skadis_nut_coupon (Autodesk Fusion 360 design; units mm, degrees)
part number: 2026-09-06-14-40-16-018
Autodesk Fusion 360 part; units mm, degrees
sketch "Plate" plane through (0, 0, 0) normal (0, 1, 0) x (1, 0, 0)
  line L0 (0, 0) -> (11, 0)
  line L1 (11, 0) -> (11, -20)
  line L2 (11, -20) -> (0, -20)
  line L3 (0, -20) -> (0, 0)
  dimension "d64" = 11
  dimension "d65" = 20
  constraint coincident L0.start L3.end
  constraint horizontal L0
  constraint horizontal L2
  constraint vertical L1
  constraint vertical L3
  measures "d64" horizontal distance of L0.start L1.end
  measures "d65" vertical distance of L0.start L1.end
extrude "Plate (1)" add sketch "Plate" along normal mid plane 33 from surface at 4.5
sketch "Screw hole" plane through (0, 0, 0) normal (0, 1, 0) x (1, 0, 0)
  line L0 (-1, -7.6) -> (12, -7.6)
  line L1 (12, -7.6) -> (12, -12.4)
  line L2 (12, -12.4) -> (-1, -12.4)
  line L3 (-1, -12.4) -> (-1, -7.6)
  dimension "d69" = 12
  dimension "d70" = 7.6
  dimension "d71" = 13
  dimension "d72" = 4.8
  constraint horizontal L0
  constraint horizontal L2
  constraint vertical L1
  constraint vertical L3
  measures "d69" horizontal distance of origin L0.end
  measures "d70" vertical distance of origin L0.end
  measures "d71" horizontal distance of L0.start L0.end
  measures "d72" vertical distance of L0.end L1.end
extrude "Screw hole (1)" cut sketch "Screw hole" along normal mid plane 16.8 from surface at 7.52
sketch "Nut cavity" plane through (0, 0, 0) normal (0, 1, 0) x (1, 0, 0)
  line L0 (5.5, -6.3) -> (8, -6.3)
  line L1 (8, -6.3) -> (8, -13.7)
  line L2 (8, -13.7) -> (5.5, -13.7)
  line L3 (5.5, -13.7) -> (5.5, -6.3)
  dimension "d76" = 8
  dimension "d77" = 6.3
  dimension "d78" = 2.5
  dimension "d79" = 7.4
  constraint horizontal L0
  constraint horizontal L2
  constraint vertical L1
  constraint vertical L3
  measures "d76" horizontal distance of origin L0.end
  measures "d77" vertical distance of origin L0.end
  measures "d78" horizontal distance of L0.start L0.end
  measures "d79" vertical distance of L0.end L1.end
extrude "Nut cavity (1)" cut sketch "Nut cavity" along normal mid plane 30.22 from surface at 2.11
equation "bracketWidth = 24.0 mm" comment "bracket width across the upright"
equation "plateHeight = 20.0 mm" comment "plate height"
equation "plateInboardExtension = 9.0 mm" comment "extra plate toward the desk centre, where the channel reaches"
equation "boardThickness = 6.0 mm" comment "measured SKADIS panel thickness"
equation "screwLength = 15.0 mm" comment "measured decorative M4 screw"
equation "screwDiameter = 4.0 mm" comment "M4 shank"
equation "screwClearance = 0.8 mm" comment "slack around the shank"
equation "screwTipClearance = 2.0 mm" comment "tip stops this short of the plate's back face"
equation "screwSlotWidth = screwDiameter + screwClearance" comment "screw relief slot height"
equation "nutAcrossFlats = 7.0 mm" comment "M4 square nut across flats"
equation "nutThickness = 2.2 mm" comment "M4 square nut thickness"
equation "nutChannelClearance = 0.4 mm" comment "slack around the nut in its channel"
equation "nutChannelHeight = nutAcrossFlats + nutChannelClearance" comment "channel height; under the nut's diagonal so it cannot turn"
equation "plateThickness = screwLength - boardThickness + screwTipClearance" comment "derived: deep enough to swallow the screw"
equation "mountTravel = 12.0 mm" comment "left-right adjustment"
equation "nutChannelLength = mountTravel + nutAcrossFlats + nutChannelClearance" comment "channel length along the plate"
equation "screwSlotLength = mountTravel + screwSlotWidth" comment "relief slot length along the plate"
equation "topMountZ = 10.0 mm" comment "top channel centre"
equation "mountOffsetY = 7.52 mm" comment "channel centre on the board's grid"
equation "slotOvershoot = 1.0 mm" comment "cuts reach past the faces they cut"
equation "nutCavityClearance = 0.3 mm" comment "slack across the nut's thickness"
equation "nutWallThickness = 3.0 mm" comment "wall in front of the nut; the screw pulls the nut against it"
equation "nutCavityDepth = nutThickness + nutCavityClearance" comment "cavity depth"
equation "d64 = plateThickness"
equation "d65 = plateHeight"
equation "d66 = plateInboardExtension / 2"
equation "d67 = bracketWidth + plateInboardExtension"
equation "d69 = plateThickness + slotOvershoot"
equation "d70 = topMountZ - screwSlotWidth / 2"
equation "d71 = plateThickness + 2 * slotOvershoot"
equation "d72 = screwSlotWidth"
equation "d73 = mountOffsetY"
equation "d74 = screwSlotLength"
equation "d76 = plateThickness - nutWallThickness"
equation "d77 = topMountZ - nutChannelHeight / 2"
equation "d78 = nutCavityDepth"
equation "d79 = nutChannelHeight"
equation "d80 = ( mountOffsetY + nutChannelLength / 2 - bracketWidth / 2 - slotOvershoot ) / 2"
equation "d81 = mountOffsetY + nutChannelLength / 2 + bracketWidth / 2 + slotOvershoot"
named bodies: "skadis_nut_coupon"
